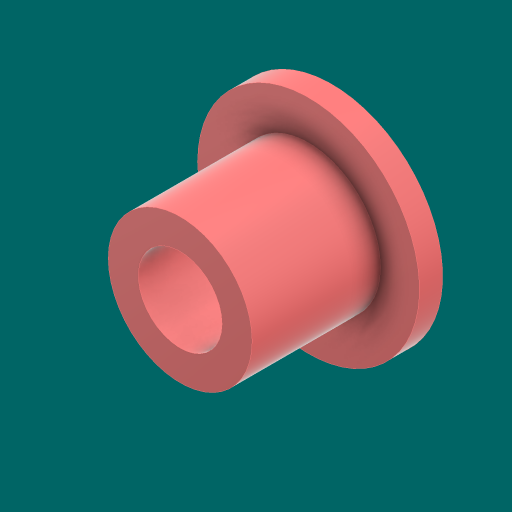
# Autodesk Inventor part: bearingsleeve
Saved by Autodesk Inventor 2023.1 (Build 271208000, 208)
## iProperties
Created: 2022-03-16
Part Number: bearingsleeve
Material: ABS Plastic
Document SubType Name: Modeling
Designer: zac-h
Density: 1.06 g/cm^3
Appearance: Smooth - Red
Author: zac-h
## iProperties of the stored document bearingsleeve_3DPrint.ipt
Created: 2022-03-17
Part Number: bearingsleeve_3DPrint
Material: Generic
Document SubType Name: Modeling
Designer: zac-h
Density: 1 g/cm^3
Appearance: Default
Author: zac-h
Autodesk Inventor part; units mm, degrees
ref_plane "YZ Plane" through (0, 0, 0) normal (1, 0, 0) x (0, 1, 0)
ref_plane "XZ Plane" through (0, 0, 0) normal (0, 1, 0) x (-1, 0, 0)
ref_plane "XY Plane" through (0, 0, 0) normal (0, 0, 1) x (1, 0, 0)
sketch "Sketch1" plane through (0, 0, 0) normal (0, 0, 1) x (1, 0, 0)
  circle A0 centre (0, 0) radius 3.925
  circle A1 centre (0, 0) radius 2.286
  dimension "d0" = 7.85
  dimension "d1" = 4.572
  constraints: 2 centre point, 2 coincident
  measures "d0" diameter of A0
  measures "d1" diameter of A1
extrude "Extrusion1" add sketch "Sketch1" against normal blind 7
sketch "Sketch2" plane through (0, 0, -7) normal (0, 0, -1) x (-1, 0, 0)
  circle A0 centre (0, 0) radius 6.05
  circle A1 centre (0, 0) radius 2.286 projected
  dimension "d4" = 12.1
  constraints: 1 centre point, 1 coincident
  measures "d4" diameter of A0
extrude "Extrusion2" add sketch "Sketch2" along normal blind 1.27
chamfer "Chamfer1" distance 0.6 angle 45 1 edges at (2.286, 0, -8.27)
body "Solid1"
